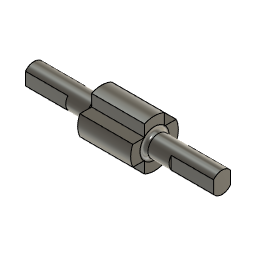
Octaped_Robot (Autodesk Fusion 360 archive; units mm, degrees)
design "drive_shaft"
Autodesk Fusion 360 part; units mm, degrees
note: some values were not read from the file. Set by a fixed rule: which face or edge a step refers to.
sketch "Sketch1" plane through (0, 0, 0) normal (1, 0, 0) x (0, 1, 0)
  line L0 (1.875, 1.875) -> (1.875, 4.0908)
  line L1 (-1.875, 4.0908) -> (-1.875, 1.875)
  line L2 (-1.875, -4.0908) -> (-1.875, -1.875)
  line L3 (1.875, -1.875) -> (1.875, -4.0908)
  line L4 (-1.875, 1.875) -> (-4.0908, 1.875)
  line L5 (-1.875, -1.875) -> (-4.0908, -1.875)
  line L6 (1.875, 1.875) -> (4.0908, 1.875)
  line L7 (1.875, -1.875) -> (4.0908, -1.875)
  arc A0 (4.0908, -1.875) -> (4.0908, 1.875) centre (0, 0) ccw
  arc A1 (-1.875, -4.0908) -> (1.875, -4.0908) centre (0, 0) ccw
  arc A2 (1.875, 4.0908) -> (-1.875, 4.0908) centre (0, 0) ccw
  arc A3 (-4.0908, 1.875) -> (-4.0908, -1.875) centre (0, 0) ccw
  constraint coincident A0.centre A1.centre
  constraint coincident L4.end A2
  constraint perpendicular L2 L5
  constraint concentric A0 A2
  constraint concentric A1 A2
  constraint concentric A2 A3
extrude "Extrude1" add sketch "Sketch1" along normal blind 15
sketch "Sketch2" plane through (15, 0, 0) normal (1, 0, 0) x (0, 1, 0)
  line L0 (1.875, 1.875) -> (1.875, 4.0908)
  arc A0 (1.875, 4.0908) -> (-1.875, 4.0908) centre (0, 0) ccw
  line L1 (-1.875, 4.0908) -> (-1.875, 1.875)
  line L2 (-1.875, 1.875) -> (-4.0908, 1.875)
  arc A1 (-4.0908, 1.875) -> (-4.0908, -1.875) centre (0, 0) ccw
  line L3 (-4.0908, -1.875) -> (-1.875, -1.875)
  line L4 (-1.875, -1.875) -> (-1.875, -4.0908)
  arc A2 (-1.875, -4.0908) -> (1.875, -4.0908) centre (0, 0) ccw
  line L5 (1.875, -4.0908) -> (1.875, -1.875)
  line L6 (1.875, -1.875) -> (4.0908, -1.875)
  arc A3 (4.0908, -1.875) -> (4.0908, 1.875) centre (0, 0) ccw
  line L7 (4.0908, 1.875) -> (1.875, 1.875)
  circle A4 centre (0, 0) radius 2
  dimension "d9" = 4
  constraint concentric A0 A4
  measures "d9" diameter of A4
extrude "Extrude2" add sketch "Sketch2" along normal blind 5 contours A4
sketch "Sketch3" plane through (20, 0, 0) normal (1, 0, 0) x (0, 1, 0)
  circle A0 centre (0, 0) radius 2
  line L0 (-1.6, 0) -> (-1.6, 1.2)
  line L1 (-1.6, 0) -> (-1.6, -1.2)
  line L2 (1.6, 0) -> (1.6, -1.2)
  line L3 (1.6, 0) -> (1.6, 1.2)
  dimension "d12" = 1.6
  constraint coincident A0 L0.end
  constraint coincident A0 L1.end
  measures "d12" distance of A0.centre L0.start
extrude "Extrude3" add sketch "Sketch3" along normal blind 10 contours A0 L0 L1 L2 L3
extrude "Extrude4" cut 1 faces at (0, 0.625, -0.625) along direction (1, 0, 0) blind 10
mirror "Mirror1" about plane through (10, 0, 0) normal (-1, 0, 0) of bodies 1 merged
extrude "Extrude5" cut 2 faces at (0, -1.6516, 0.3199) (0, 1.8121, 0.2345) along direction (1, 0, 0) blind 1
extrude "Extrude6" cut 2 faces at (20, 1.8121, 0.2345) (20, -1.6516, 0.3199) along direction (-1, 0, 0) blind 1
fillet "Fillet3" radius 0.75 1 edges at (15, -1.8647, 0.7232)
extrude "Extrude7" cut 1 faces at (30, -0.5956, 0.4718) along direction (-1, 0, 0) blind 7
extrude "Extrude8" cut 1 faces at (-10, -0.5956, 0.4718) along direction (1, 0, 0) blind 7
extrude "Extrude9" add 2 faces at (1, -1.6516, 0.3199) (1, 1.8121, 0.0634) along direction (-1, 0, 0) blind 0.75
fillet "Fillet5" radius 0.75 1 edges at (5, -1.8647, 0.7232)
extrude "Extrude10" add 1 faces at (-3, -0.5956, 0.4718) along direction (-1, 0, 0) blind 0.75
extrude "Extrude11" add 2 faces at (19, -1.6516, 0.3199) (19, 1.6469, -0.3282) along direction (1, 0, 0) blind 0.75
extrude "Extrude12" add 1 faces at (23, -0.5956, 0.4718) along direction (1, 0, 0) blind 0.75
extrude "Extrude13" add 1 faces at (-3.75, -0.5956, 0.4718) along direction (-1, 0, 0) blind 4
extrude "Extrude14" add 1 faces at (23.75, -0.5956, 0.4718) along direction (1, 0, 0) blind 4
